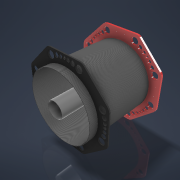
# Autodesk Inventor part: PrimaryMirror
Saved by Autodesk Inventor 2022 (Build 260153000, 153)
## iProperties
Created: 2021-05-06
Part Number: PrimaryMirror
Material: Generic
Document SubType Name: Modeling
Designer: Mick Veldhuis
Density: 1 g/cm^3
Appearance: Default
Mass: 10922.3 g
Surface Area: 20818.6 cm^2
Volume: 10922.3 cm^3
Author: Mick Veldhuis
Autodesk Inventor part; units mm, degrees
ref_plane "YZ Plane" through (0, 0, 0) normal (1, 0, 0) x (0, 1, 0)
ref_plane "XZ Plane" through (0, 0, 0) normal (0, 1, 0) x (-1, 0, 0)
ref_plane "XY Plane" through (0, 0, 0) normal (0, 0, 1) x (1, 0, 0)
sketch "Sketch1" plane through (0, 0, 0) normal (0, 0, 1) x (1, 0, 0)
  line L0 (-264, 109.3524) -> (-109.3524, 264)
  line L1 (-109.3524, 264) -> (109.3524, 264)
  line L2 (109.3524, 264) -> (264, 109.3524)
  line L3 (264, 109.3524) -> (264, -109.3524)
  line L4 (264, -109.3524) -> (109.3524, -264)
  line L5 (109.3524, -264) -> (-109.3524, -264)
  line L6 (-109.3524, -264) -> (-264, -109.3524)
  line L7 (-264, -109.3524) -> (-264, 109.3524)
  point P0 (0, 0)
  point P1 (0, 0)
  constraints: 16 end point, 1 coincident, 17 other
extrude "Extrusion1" add sketch "Sketch1" against normal blind 14
sketch "Backplate" plane through (0, 0, 0) normal (0, 0, 1) x (1, 0, 0)
  circle A0 centre (0, 0) radius 203
  circle A1 centre (0, 0) radius 200
  circle A2 centre (-170, 170) radius 9
  circle A3 centre (-186, 150) radius 11
  circle A4 centre (-150, 186) radius 11
  circle A5 centre (-124, 204) radius 14
  circle A6 centre (-204, 124) radius 14
  circle A7 centre (-90, 226) radius 21
  circle A8 centre (-226, 90) radius 21
  line L0 (0, 281) -> (0, -280.0278) construction
  line L1 (-109.3524, 264) -> (109.3524, 264) construction
  line L2 (-280, 0) -> (280, 0) construction
  circle A9 centre (-226, -90) radius 21
  circle A10 centre (-204, -124) radius 14
  circle A11 centre (-186, -150) radius 11
  circle A12 centre (-170, -170) radius 9
  circle A13 centre (-150, -186) radius 11
  circle A14 centre (-124, -204) radius 14
  circle A15 centre (-90, -226) radius 21
  circle A16 centre (226, 90) radius 21
  circle A17 centre (204, 124) radius 14
  circle A18 centre (186, 150) radius 11
  circle A19 centre (170, 170) radius 9
  circle A20 centre (150, 186) radius 11
  circle A21 centre (124, 204) radius 14
  circle A22 centre (90, 226) radius 21
  line L3 (109.3524, 264) -> (-109.3524, 264) construction
  circle A23 centre (204, -124) radius 14
  circle A24 centre (186, -150) radius 11
  circle A25 centre (170, -170) radius 9
  circle A26 centre (150, -186) radius 11
  circle A27 centre (226, -90) radius 21
  circle A28 centre (124, -204) radius 14
  circle A29 centre (90, -226) radius 21
  circle A30 centre (0, 0) radius 50
  circle A31 centre (0, 0) radius 52
  circle A32 centre (0, 0) radius 57
  circle A33 centre (0, 0) radius 195
  point P0 (-109.3524, -264)
  point P1 (109.3524, -264)
  constraints: 34 centre point, 31 symmetric about line, 14 coincident, 6 end point, 1 horizontal, 1 perpendicular, 21 other
extrude "Extrusion2" add sketch "Backplate" along normal blind 416 contours A0
extrude "Extrusion3" add sketch "Backplate" along normal blind 440 contours A31
extrude "Extrusion4" add sketch "Backplate" along normal blind 50 contours A33
hole "Hole1" at (-226, -90, 0) at (-226, 90, 0) at (-90, 226, 0) at (90, 226, 0) at (226, 90, 0) at (226, -90, 0) at (90, -226, 0) at (-90, -226, 0) direction (0, 0, -1) diameter 42 end through all
hole "Hole2" at (-204, 124, 0) at (-124, 204, 0) at (124, 204, 0) at (204, 124, 0) at (-124, -204, 0) at (-204, -124, 0) direction (0, 0, -1) diameter 28 end through all
hole "Hole3" at (-90, 226, 0) at (-150, 186, 0) at (-150, -186, 0) at (150, -186, 0) at (150, 186, 0) at (-186, 150, 0) at (186, 150, 0) at (-186, -150, 0) at (186, -150, 0) direction (0, 0, -1) diameter 22 end through all
hole "Hole4" at (124, -204, 0) at (204, -124, 0) direction (0, 0, -1) diameter 28 end through all
hole "Hole5" at (-170, -170, 0) at (-170, 170, 0) at (170, 170, 0) at (170, -170, 0) direction (0, 0, -1) diameter 18 end through all
fillet "Fillet1" radius 40 8 edges at (264, -109.3524, -7) (109.3524, -264, -7) (-109.3524, -264, -7) (-264, -109.3524, -7) (-264, 109.3524, -7) (-109.3524, 264, -7) (109.3524, 264, -7) (264, 109.3524, -7)
ref_plane "Work Plane1" through (0, 0, 360) normal (0, 0, 1) x (1, 0, 0)
sketch "Sketch3" plane through (0, 0, 360) normal (0, 0, 1) x (1, 0, 0)
  line L0 (264, 92.7838) -> (264, -92.7838) projected
  line L1 (264, -109.3524) -> (109.3524, -264)
  line L2 (109.3524, -264) -> (-109.3524, -264)
  line L3 (-109.3524, -264) -> (-264, -109.3524)
  line L4 (-264, -109.3524) -> (-264, 109.3524)
  line L5 (-264, 109.3524) -> (-109.3524, 264)
  line L6 (-109.3524, 264) -> (109.3524, 264)
  line L7 (109.3524, 264) -> (264, 109.3524)
  line L8 (264, 109.3524) -> (264, -109.3524)
  point P0 (0, 0)
  point P1 (0, 0)
  point P2 (264, 0)
  point P3 (264, -92.7838)
  constraints: 16 end point, 2 midpoint, 1 coincident, 17 other
extrude "Extrusion5" add sketch "Sketch3" along normal blind 8
fillet "Fillet2" radius 40 8 edges at (-109.3524, 264, 364) (-264, 109.3524, 364) (-264, -109.3524, 364) (-109.3524, -264, 364) (109.3524, -264, 364) (264, -109.3524, 364) (264, 109.3524, 364) (109.3524, 264, 364)
ref_plane "Work Plane2" through (0, 0, 368) normal (0, 0, 1) x (1, 0, 0)
sketch "Frontplate" plane through (0, 0, 368) normal (0, 0, 1) x (1, 0, 0)
  circle A0 centre (-226, 90) radius 21
  circle A1 centre (-90, 226) radius 21
  line L0 (0, 321) -> (0, -319) construction
  line L1 (-319, 0) -> (310, 0) construction
  circle A2 centre (-90, -226) radius 21
  circle A3 centre (-226, -90) radius 21
  circle A4 centre (90, 226) radius 21
  circle A5 centre (226, 90) radius 21
  circle A6 centre (90, -226) radius 21
  circle A7 centre (226, -90) radius 21
  circle A8 centre (0, 0) radius 200
  circle A9 centre (0, 0) radius 52
  circle A10 centre (0, 0) radius 200
  circle A11 centre (0, 0) radius 213
  circle A12 centre (238, -52) radius 14
  circle A13 centre (242, -24) radius 11
  circle A14 centre (244, 0) radius 9
  circle A15 centre (242, 24) radius 11
  circle A16 centre (238, 52) radius 14
  circle A17 centre (-238, -52) radius 14
  circle A18 centre (-242, -24) radius 11
  circle A19 centre (-244, 0) radius 9
  circle A20 centre (-242, 24) radius 11
  circle A21 centre (-238, 52) radius 14
  circle A22 centre (-52.0028, -238.0327) radius 14
  circle A23 centre (-24.0028, -242.0327) radius 11
  circle A24 centre (0, -244) radius 9
  circle A25 centre (23.9972, -242.0327) radius 11
  circle A26 centre (51.9972, -238.0327) radius 14
  circle A27 centre (51.9972, 237.9673) radius 14
  circle A28 centre (23.9972, 241.9673) radius 11
  circle A29 centre (0, 244) radius 9
  circle A30 centre (-24.0028, 241.9673) radius 11
  circle A31 centre (-52.0028, 237.9673) radius 14
  constraints: 32 centre point, 11 symmetric about line, 4 coincident, 4 end point, 2 point on line, 1 concentric, 1 horizontal, 1 vertical, 11 other
extrude "Extrusion6" cut sketch "Frontplate" against normal up to next contours A8
sketch "Sketch5" plane through (0, 0, 368) normal (0, 0, 1) x (1, 0, 0)
  circle A0 centre (0, 0) radius 50
  constraints: 1 centre point, 1 coincident
extrude "Extrusion7" cut sketch "Sketch5" against normal up to next
hole "Hole6" at (-90, 226, 368) at (90, 226, 368) at (-226, 90, 368) at (-226, -90, 368) at (90, -226, 368) at (-90, -226, 368) at (226, -90, 368) at (226, 90, 368) direction (0, 0, -1) diameter 42 end through all
hole "Hole7" at (-52.0028, 237.9673, 368) at (51.9972, 237.9673, 368) at (238, 52, 368) at (238, -52, 368) at (-238, 52, 368) at (-238, -52, 368) at (51.9972, -238.0327, 368) at (-52.0028, -238.0327, 368) direction (0, 0, -1) diameter 28 depth 8 tip angle 118
hole "Hole8" at (23.9972, -242.0327, 368) at (-24.0028, -242.0327, 368) at (-242, -24, 368) at (-242, 24, 368) at (242, 24, 368) at (242, -24, 368) at (23.9972, 241.9673, 368) at (-24.0028, 241.9673, 368) direction (0, 0, -1) diameter 22 depth 8 tip angle 118
hole "Hole9" at (-244, 0, 368) at (0, -244, 368) at (244, 0, 368) at (0, 244, 368) direction (0, 0, -1) diameter 18 depth 8 tip angle 118
sketch "Sketch6" plane through (0, 0, -14) normal (0, 0, -1) x (-1, 0, 0)
  line L0 (-36, 251) -> (36, 251) construction
  line L1 (36, 251) -> (36, 229) construction
  line L2 (36, 229) -> (-36, 229) construction
  line L3 (-36, 229) -> (-36, 251) construction
  line L4 (-36, 251) -> (36, 229) construction
  line L5 (36, 251) -> (-36, 229) construction
  line L6 (0, -280) -> (0, 301) construction
  line L7 (-282, 0) -> (279, 0) construction
  line L8 (-36, -251) -> (36, -251) construction
  line L9 (36, -251) -> (36, -229) construction
  line L10 (36, -229) -> (-36, -229) construction
  line L11 (-36, -229) -> (-36, -251) construction
  line L12 (-36, -251) -> (36, -229) construction
  line L13 (36, -251) -> (-36, -229) construction
  line L14 (-251, 36) -> (-229, 36) construction
  line L15 (-229, 36) -> (-229, -36) construction
  line L16 (-229, -36) -> (-251, -36) construction
  line L17 (-251, -36) -> (-251, 36) construction
  line L18 (-251, 36) -> (-229, -36) construction
  line L19 (-229, 36) -> (-251, -36) construction
  line L20 (251, 36) -> (229, 36) construction
  line L21 (229, 36) -> (229, -36) construction
  line L22 (229, -36) -> (251, -36) construction
  line L23 (251, -36) -> (251, 36) construction
  line L24 (251, 36) -> (229, -36) construction
  line L25 (229, 36) -> (251, -36) construction
  point P0 (0, 0)
  point P1 (0, 240)
  point P2 (-28, 240)
  point P3 (28, 240)
  point P4 (0, -240)
  point P5 (-28, -240)
  point P6 (28, -240)
  point P7 (-240, 0)
  point P8 (-240, 28)
  point P9 (-240, -28)
  point P10 (240, 0)
  point P11 (240, 28)
  point P12 (240, -28)
  constraints: 52 end point, 14 symmetric about line, 8 midpoint, 4 parallel, 3 horizontal, 2 perpendicular, 1 point on line, 1 vertical
hole "Hole10" at (28, 240, -14) at (-28, -240, -14) at (28, -240, -14) at (240, 28, -14) at (240, -28, -14) at (-240, -28, -14) at (-240, 28, -14) at (-28, 240, -14) direction (0, 0, 1) diameter 3.242 depth 14 thread size "M4x0.7" class "6H" standard "ISO Metric profile"
sketch "Sketch7" plane through (-121.0681, 252.2843, -14) normal (-0.7071068, 0.7071068, 0) x (-0.7071068, -0.7071068, 0)
  line L0 (0, 0) -> (0, 14) projected
  line L1 (185.5677, 14) -> (185.5677, 0) projected
  point P0 (92.7838, 14)
  point P1 (93, 7)
sketch "Sketch8" plane through (-252.2843, 121.0681, 360) normal (-0.7071068, 0.7071068, 0) x (-0.7071068, -0.7071068, 0)
  point P0 (-92.7838, -360)
  point P1 (-92.7838, 4)
hole "Hole11" at (-186.6762, 186.6762, 364) direction (0.7071068, -0.7071068, 0) diameter 4.917 depth 30 tip angle 118 thread size "M6x1" class "6H" standard "ISO Metric profile"
hole "Hole12" at (-186.829, 186.5233, -7) direction (0.7071068, -0.7071068, 0) diameter 4.917 depth 30 tip angle 118 thread size "M6x1" class "6H" standard "ISO Metric profile"
body "Solid1"
